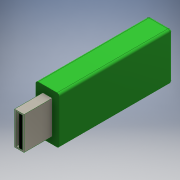
# Autodesk Inventor part: USB_Stick
Saved by Autodesk Inventor 2016 (Build 200138000, 138)
## iProperties
Created: 2017-07-18
Part Number: USB_Stick
Material: ABS Plastic
Document SubType Name: Modeling
Designer: bobbyl
Density: 1.06 g/cm^3
Appearance: Smooth - Dark Forest Green
Author: bobbyl
Autodesk Inventor part; units mm, degrees
ref_plane "YZ Plane" through (0, 0, 0) normal (1, 0, 0) x (0, 1, 0)
ref_plane "XZ Plane" through (0, 0, 0) normal (0, 1, 0) x (-1, 0, 0)
ref_plane "XY Plane" through (0, 0, 0) normal (0, 0, 1) x (1, 0, 0)
sketch "Sketch1" plane through (0, 0, 0) normal (0, 1, 0) x (-1, 0, 0)
  line L0 (12.5, 25) -> (-12.5, 25)
  line L1 (-12.5, 25) -> (-12.5, -25)
  line L2 (-12.5, -25) -> (12.5, -25)
  line L3 (12.5, -25) -> (12.5, 25)
  line L4 (17.5, 0) -> (-17.5, 0) projected
  line L5 (0, -35) -> (0, 35) projected
  point P0 (0, 0)
  point P1 (12.5, 0)
  point P2 (0, -25)
  dimension "d0" = 50
  dimension "d1" = 25
  constraints: 8 end point, 2 midpoint, 2 parallel, 2 point on line, 1 horizontal, 1 perpendicular
  measures "d0" distance of L2.end L0.start
  measures "d1" distance of L0.start L0.end
extrude "Extrusion1" add sketch "Sketch1" along normal mid plane 120
sketch "Sketch2" plane through (0, -60, 0) normal (0, -1, 0) x (1, 0, 0)
  line L0 (-12.5, -25) -> (12.5, -25) projected
  line L1 (12.5, -25) -> (12.5, 25) projected
  line L2 (12.5, 25) -> (-12.5, 25) projected
  line L3 (-12.5, 25) -> (-12.5, -25) projected
  line L4 (5, 17.5) -> (5, -17.5)
  line L5 (5, -17.5) -> (-5, -17.5)
  line L6 (-5, -17.5) -> (-5, 17.5)
  line L7 (-5, 17.5) -> (5, 17.5)
  point P0 (0, 0)
  dimension "d4" = 10
  constraints: 8 end point, 3 other
  measures "d4" distance between parallel lines of L4 L6
extrude "Extrusion2" add sketch "Sketch2" along normal blind 30 contours L4 L5 L6 L7
sketch "Sketch3" plane through (0, -90, 0) normal (0, -1, 0) x (1, 0, 0)
  line L0 (5, -17.5) -> (5, 17.5) projected
  line L1 (5, 17.5) -> (-5, 17.5) projected
  line L2 (-5, 17.5) -> (-5, -17.5) projected
  line L3 (-5, -17.5) -> (5, -17.5) projected
  line L4 (-3.5, -16) -> (0, -16)
  line L5 (0, -16) -> (0, 16)
  line L6 (0, 16) -> (-3.5, 16)
  line L7 (-3.5, 16) -> (-3.5, -16)
  line L8 (-17.5, 0) -> (17.5, 0) projected
  line L9 (0, -35) -> (0, 35) projected
  point P0 (0, 0)
  point P1 (-3.5, 0)
  dimension "d7" = 1.5
  dimension "d8" = 1.5
  constraints: 8 end point, 2 parallel, 1 collinear, 1 horizontal, 1 midpoint, 1 perpendicular, 1 point on line
  measures "d7" distance between parallel lines of L7 L2
  measures "d8" distance between parallel lines of L1 L6
extrude "Extrusion3" cut sketch "Sketch3" against normal blind 30 contours L8 L7 L6 L5 | L5 L4 L7 L8
sketch "Sketch4" plane through (-5, -60, -17.5) normal (-1, 0, 0) x (0, 0, 1)
  line L0 (0, 0) -> (35, 0) projected
  line L1 (0, 0) -> (0, -30) projected
  line L2 (35, -30) -> (0, -30) projected
  line L3 (35, 0) -> (35, -30) projected
  line L4 (17.5, -60) -> (17.5, 150) projected
  line L5 (5, -8) -> (11.5, -8)
  line L6 (11.5, -8) -> (11.5, -14.5)
  line L7 (11.5, -14.5) -> (5, -14.5)
  line L8 (5, -14.5) -> (5, -8)
  line L9 (30, -8) -> (23.5, -8)
  line L10 (23.5, -8) -> (23.5, -14.5)
  line L11 (23.5, -14.5) -> (30, -14.5)
  line L12 (30, -14.5) -> (30, -8)
  point P0 (17.5, 60)
  dimension "d11" = 6.5
  dimension "d12" = 6
  dimension "d13" = 8
  constraints: 16 end point, 4 symmetric about line, 2 parallel, 2 perpendicular, 1 horizontal
  measures "d11" distance of L6.end L7.end
  measures "d12" distance between parallel lines of L4 L6
  measures "d13" distance between parallel lines of L5 L0
extrude "Extrusion4" cut sketch "Sketch4" against normal blind 1 contours L5 L6 L7 L8 | L12 L11 L10 L9
fillet "Fillet1" radius 2.5 8 edges at (-12.5, 0, 25) (-12.5, 0, -25) (12.5, 0, 25) (12.5, 0, -25) (0, 60, 25) (-12.5, 60, 0) (0, 60, -25) (12.5, 60, 0)
sketch "Sketch5" plane through (0, -90, 0) normal (0, -1, 0) x (1, 0, 0)
  line L0 (0, -16) -> (-3.5, -16) projected
  line L1 (-3.5, -16) -> (-3.5, 16) projected
  line L2 (-3.5, 16) -> (0, 16) projected
  line L3 (0, 16) -> (0, -16) projected
  line L4 (5, -17.5) -> (5, 17.5) projected
  line L5 (5, 17.5) -> (-5, 17.5) projected
  line L6 (-5, 17.5) -> (-5, -17.5) projected
  line L7 (-5, -17.5) -> (5, -17.5) projected
  line L8 (0, -16) -> (3.5, -16)
  line L9 (3.5, -16) -> (3.5, 16)
  line L10 (3.5, 16) -> (0, 16)
  line L11 (0, 16) -> (0, -16)
  point P0 (0, 0)
  dimension "d17" = 1.5
  dimension "d18" = 1.5
  constraints: 8 end point, 2 parallel, 1 horizontal, 1 perpendicular
  measures "d17" distance between parallel lines of L4 L9
  measures "d18" distance between parallel lines of L5 L10
extrude "Extrusion5" cut sketch "Sketch5" against normal blind 0.01 contours L3 L10 L9 L8
body "Solid1"
